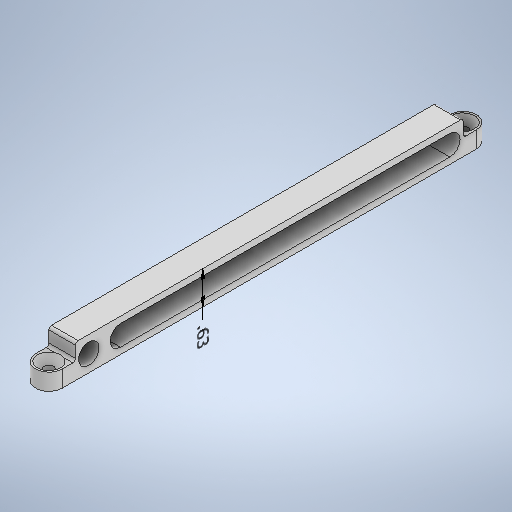
# Autodesk Inventor part: Scissor Base
Saved by Autodesk Inventor 2025.1 (Build 291241000, 241)
## iProperties
Created: 2025-10-25
Part Number: Scissor Base
Material: Generic
Document SubType Name: Modeling
Designer: benja
Density: 1 g/cm^3
Appearance: Default
Author: benja
Autodesk Inventor part; units mm, degrees
ref_plane "YZ Plane" through (0, 0, 0) normal (1, 0, 0) x (0, 1, 0)
ref_plane "XZ Plane" through (0, 0, 0) normal (0, 1, 0) x (-1, 0, 0)
ref_plane "XY Plane" through (0, 0, 0) normal (0, 0, 1) x (1, 0, 0)
sketch "Sketch1" plane through (0, 0, 0) normal (0, 1, 0) x (-1, 0, 0)
  line L0 (0, 0) -> (0, -197.866) construction
  line L1 (-6.35, 0) -> (-6.35, -197.866)
  line L2 (6.35, -197.866) -> (6.35, 0)
  arc A0 (6.35, 0) -> (-6.35, 0) centre (0, 0) ccw
  arc A1 (-6.35, -197.866) -> (6.35, -197.866) centre (0, -197.866) ccw
  circle A2 centre (0, 0) radius 2.2987
  line L3 (0, -98.933) -> (6.35, -98.933)
  circle A3 centre (0, -197.866) radius 2.2987
  line L4 (-6.35, 6.35) -> (6.35, 6.35)
  line L5 (6.35, 6.35) -> (6.35, -6.35)
  line L6 (6.35, -6.35) -> (-6.35, -6.35)
  line L7 (-6.35, -6.35) -> (-6.35, 6.35)
  line L8 (-6.35, 6.35) -> (6.35, -6.35) construction
  line L9 (6.35, 6.35) -> (-6.35, -6.35) construction
  line L10 (-6.35, -204.216) -> (6.35, -204.216)
  line L11 (6.35, -204.216) -> (6.35, -191.516)
  line L12 (6.35, -191.516) -> (-6.35, -191.516)
  line L13 (-6.35, -191.516) -> (-6.35, -204.216)
  line L14 (-6.35, -204.216) -> (6.35, -191.516) construction
  line L15 (6.35, -204.216) -> (-6.35, -191.516) construction
  dimension "d0" = 197.866
  dimension "d1" = 12.7
  dimension "d2" = 4.5974
  dimension "d3" = 12.7
  dimension "d4" = 12.7
  dimension "d5" = 12.7
  dimension "d6" = 12.7
  constraints: 34 end point, 6 midpoint, 5 parallel, 4 centre point, 4 point on circle, 4 tangent, 2 horizontal, 2 perpendicular, 1 coincident, 1 symmetric about line, 1 vertical, 1 other
  measures "d0" distance of L0.start L0.end
  measures "d1" diameter of A1
  measures "d2" diameter of A2
  measures "d3" distance of L5.end L6.end
  measures "d4" distance of L4.end L5.end
  measures "d5" distance of L12.end L11.end
  measures "d6" distance of L11.end L10.end
extrude "Extrusion1" add sketch "Sketch1" along normal blind 12.7 contours L6 L2 L12 L1
extrude "Extrusion2" add sketch "Sketch1" along normal blind 6.35 contours A0 L2 L6 L1 | L12 L2 A1 L1
chamfer "Chamfer1" distance 3.175 angle 45 2 edges at (2.2987, 6.35, 0) (2.2987, 6.35, -197.866)
sketch "Sketch2" plane through (6.35, 12.7, -6.35) normal (1, 0, 0) x (0, 0, -1)
  line L0 (-6.35, -12.7) -> (191.516, -12.7) projected
  line L1 (191.516, -12.7) -> (191.516, -6.35) projected
  line L2 (185.166, -6.35) -> (191.516, -6.35) projected
  line L3 (185.166, -6.35) -> (185.166, 0) projected
  line L4 (0, 0) -> (185.166, 0) projected
  line L5 (0, -6.35) -> (0, 0) projected
  line L6 (-6.35, -6.35) -> (0, -6.35) projected
  line L7 (-6.35, -12.7) -> (-6.35, -6.35) projected
  line L8 (0, -6.35) -> (0, -12.7)
  line L9 (185.166, -6.35) -> (185.166, -12.7)
  line L10 (0, -6.35) -> (6.3485, -6.35)
  line L11 (185.166, -6.35) -> (178.816, -6.35)
  circle A0 centre (6.3485, -6.35) radius 4.8895
  line L12 (178.816, -6.35) -> (21.4671, -6.35) construction
  line L13 (178.816, -1.4605) -> (21.4671, -1.4605)
  line L14 (21.4671, -11.2395) -> (178.816, -11.2395)
  arc A1 (178.816, -11.2395) -> (178.816, -1.4605) centre (178.816, -6.35) ccw
  arc A2 (21.4671, -1.4605) -> (21.4671, -11.2395) centre (21.4671, -6.35) ccw
  point P0 (100.1415, -6.35)
  dimension "d14" = 6.35
  dimension "d15" = 9.779
  dimension "d16" = 9.779
  constraints: 16 end point, 4 point on circle, 4 tangent, 3 centre point, 2 horizontal, 2 parallel, 2 perpendicular, 2 point on line, 1 coincident, 1 midpoint
  measures "d14" distance of L2.start L11.end
  measures "d15" diameter of A0
  measures "d16" diameter of A2
extrude "Extrusion3" cut sketch "Sketch2" against normal blind 33.3375 contours A0 | A1 L14 A2 L13
sketch "Sketch3" plane through (6.35, 0, 0) normal (1, 0, 0) x (0, 0, -1)
  circle A0 centre (12.6985, 6.35) radius 4.8895 projected
  arc A1 (27.8171, 11.2395) -> (27.8171, 1.4605) centre (27.8171, 6.35) ccw projected
  line L0 (27.8171, 11.2395) -> (185.166, 11.2395) projected
  arc A2 (185.166, 1.4605) -> (185.166, 11.2395) centre (185.166, 6.35) ccw projected
  line L1 (185.166, 1.4605) -> (27.8171, 1.4605) projected
  arc A3 (27.8171, 11.2395) -> (27.8171, 1.4605) centre (27.8171, 6.35) ccw projected
  circle A4 centre (12.6985, 6.35) radius 4.8895 projected
  line L2 (6.35, 6.35) -> (6.35, 12.7) projected
  line L3 (0, 6.35) -> (6.35, 6.35) projected
  line L4 (0, 0) -> (0, 6.35) projected
  line L5 (0, 0) -> (197.866, 0) projected
  line L6 (197.866, 0) -> (197.866, 6.35) projected
  line L7 (191.516, 6.35) -> (197.866, 6.35) projected
  line L8 (191.516, 6.35) -> (191.516, 12.7) projected
  line L9 (6.35, 12.7) -> (191.516, 12.7) projected
  line L10 (12.6985, 6.35) -> (134.6504, 128.3019) construction
  line L11 (17.1887, 1.8599) -> (139.1405, 123.8118)
  line L12 (130.1603, 132.792) -> (8.2084, 10.8401)
  arc A5 (8.2084, 10.8401) -> (17.1887, 1.8599) centre (12.6985, 6.35) ccw
  arc A6 (139.1405, 123.8118) -> (130.1603, 132.792) centre (134.6504, 128.3019) ccw
  line L13 (12.6985, 6.35) -> (185.1645, 6.35) construction
  line L14 (73.6745, 67.3259) -> (134.6504, 6.35)
  line L15 (134.6504, 6.35) -> (12.6985, 128.3019) construction
  line L16 (139.1405, 10.8401) -> (17.1887, 132.792)
  line L17 (8.2084, 123.8118) -> (130.1603, 1.8599)
  arc A7 (130.1603, 1.8599) -> (139.1405, 10.8401) centre (134.6504, 6.35) ccw
  arc A8 (17.1887, 132.792) -> (8.2084, 123.8118) centre (12.6985, 128.3019) ccw
  circle A9 centre (73.6745, 67.3259) radius 4.8895
  dimension "d20" = 172.466
  dimension "d21" = 45
  dimension "d22" = 12.7
  dimension "d23" = 172.466
  dimension "d24" = 12.7
  dimension "d25" = 9.779
  dimension "d26" = 9.779
  constraints: 20 end point, 8 point on circle, 8 tangent, 5 centre point, 2 midpoint, 2 parallel, 1 coincident, 1 equal length, 1 horizontal, 1 point on line
  measures "d20" distance of L10.start L10.end
  measures "d21" angle of L13 L10
  measures "d22" diameter of A6
  measures "d23" distance of L14.end L15.end
  measures "d24" diameter of A8
  measures "d25" diameter of A9
  measures "d26" diameter of A4
extrude "Extrusion4" add sketch "Sketch1" against normal blind 1.5875 contours A0 L2 L6 L1 | L6 L2 L12 L1 | L12 L2 A1 L1
sketch "Sketch4" plane through (0, 12.7, 0) normal (0, 1, 0) x (1, 0, 0)
  line L0 (6.35, 6.35) -> (6.35, 191.516) projected
  line L1 (-6.35, 191.516) -> (-6.35, 6.35) projected
  line L2 (-6.35, 6.35) -> (6.35, 6.35) projected
  line L3 (6.35, 191.516) -> (-6.35, 191.516) projected
  point P0 (0, 0)
extrude "Extrusion5" add sketch "Sketch4" along normal blind 1.5875
fillet "Fillet2" radius 1.27 4 edges at (0, 14.2875, -191.516) (0, 6.35, -191.516) (0, 6.35, -6.35) (0, 14.2875, -6.35)
body "Solid1"
